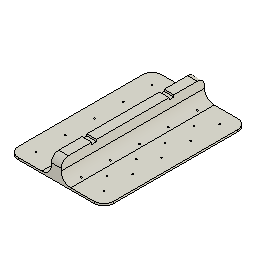
Tempeh-mould-10x15 (Autodesk Fusion 360 archive; units mm, degrees)
design "Tempeh-mould-lid-10x15"
Autodesk Fusion 360 part; units mm, degrees
sketch "sketch-footprint-box" plane through (0, 0, 0) normal (0, 0, 1) x (1, 0, 0)
  line L0 (-50, 75) -> (50, 75) construction
  line L1 (50, 75) -> (50, -75) construction
  line L2 (50, -75) -> (-50, -75) construction
  line L3 (-50, -75) -> (-50, 75) construction
  line L4 (-50, 75) -> (50, -75) construction
  line L5 (50, 75) -> (-50, -75) construction
  line L6 (49.25, 74.25) -> (-49.25, 74.25)
  line L7 (-49.25, 74.25) -> (-49.25, -74.25)
  line L8 (-49.25, -74.25) -> (49.25, -74.25)
  line L9 (49.25, -74.25) -> (49.25, 74.25)
  line L10 (49.25, 74.25) -> (-49.25, -74.25) construction
  line L11 (-49.25, 74.25) -> (49.25, -74.25) construction
  dimension "width" = 100
  dimension "length" = 150
  dimension "d104" = 0.75
  dimension "d105" = 0.75
  constraint horizontal L0
  constraint vertical L1
  constraint horizontal L2
  constraint vertical L3
  constraint midpoint L5 origin
  constraint horizontal L6
  constraint perpendicular L6 L7
  constraint parallel L6 L8
  constraint parallel L7 L9
  constraint coincident L10 origin
  constraint coincident L11 origin
  measures "width" distance of L0.start L0.end
  measures "length" distance of L0.start L2.end
  measures "d104" distance of L0 L6
  measures "d105" distance of L3 L7
extrude "Extrude1" add sketch "sketch-footprint-box" along normal blind 2
sketch "Sketch-lid" plane through (0, 0, 2) normal (0, 0, 1) x (-1, 0, 0)
  line L0 (5, -74.25) -> (-5, -74.25)
  line L1 (-5, -74.25) -> (-5, 74.25)
  line L2 (-5, 74.25) -> (5, 74.25)
  line L3 (5, 74.25) -> (5, -74.25)
  line L4 (5, -74.25) -> (-5, 74.25) construction
  line L5 (-5, -74.25) -> (5, 74.25) construction
  line L6 (-49.25, 74.25) -> (-49.25, -74.25)
  line L7 (-49.25, -74.25) -> (49.25, -74.25)
  line L8 (49.25, -74.25) -> (49.25, 74.25)
  line L9 (49.25, 74.25) -> (-49.25, 74.25)
  dimension "handle_width" = 10
  constraint horizontal L0
  constraint vertical L1
  constraint horizontal L2
  constraint vertical L3
  constraint midpoint L5 origin
  constraint coincident L1.end L9
  measures "handle_width" distance of L0.start L0.end
extrude "Extrude2" add sketch "Sketch-lid" along normal blind 20 contours L0 L1 L2 L3 L7 L9
extrude "Extrude8" add 1 faces at (16.4167, 24.75, 0) along direction (0, 0, -1) blind 0.0001
draft "Draft18" angle 0 neutral plane through (0, 0, 22) pull (0, 0, 1) 1 faces at (-5, -24.75, 8.6667)
draft "Draft19" angle 0 neutral plane through (0, 0, 22) pull (0, 0, 1) 1 faces at (5, 24.75, 8.6667)
draft "Draft20" angle 0 neutral plane through (0, 0, 22) pull (0, 0, 1) 1 faces at (-1.6667, -74.25, 8.6667)
draft "Draft21" angle 0 neutral plane through (0, 0, 22) pull (0, 0, 1) 1 faces at (1.6667, 74.25, 15.3333)
draft "Draft22" angle 0 neutral plane through (0, 0, 2) pull (0, 0, 1) 1 faces at (49.25, 24.75, 0.6666)
draft "Draft23" angle 0 neutral plane through (0, 0, 2) pull (0, 0, 1) 1 faces at (-49.25, 24.75, 1.3333)
fillet "Fillet5" radius 10 4 edges at (49.25, -74.25, 0.9999) (49.25, 74.25, 1) (-49.25, 74.25, 1) (-49.25, -74.25, 1)
fillet "Fillet6" radius 10 2 edges at (-5, 0, 2) (5, 0, 2)
fillet "Fillet7" radius 7.5 2 edges at (0, -74.25, 22) (0, 74.25, 22)
sketch "Sketch-notches-handle" plane through (0, 0, 22) normal (0, 0, 1) x (-1, 0, 0)
  line L0 (5, -66.75) -> (5, 66.75)
  line L1 (-5, 66.75) -> (-5, -66.75)
  line L2 (5, -42.5) -> (-5, -42.5)
  line L3 (-5, -42.5) -> (-5, -37.5)
  line L4 (-5, -37.5) -> (5, -37.5)
  line L5 (5, -37.5) -> (5, -42.5)
  line L6 (5, 37.5) -> (-5, 37.5)
  line L7 (-5, 37.5) -> (-5, 42.5)
  line L8 (-5, 42.5) -> (5, 42.5)
  line L9 (5, 42.5) -> (5, 37.5)
  line L10 (5, -37.5) -> (-5, 37.5) construction
  line L11 (-5, -37.5) -> (5, 37.5) construction
  line L12 (5, -37.5) -> (-5, -42.5) construction
  line L13 (5, -42.5) -> (-5, -37.5) construction
  line L14 (5, 42.5) -> (-5, 37.5) construction
  line L15 (-5, 42.5) -> (5, 37.5) construction
  circle A0 centre (0, -40) radius 0.75
  circle A1 centre (0, 40) radius 0.75
  line L16 (0, -37.5) -> (0, 0) construction
  line L17 (0, 0) -> (0, 37.5) construction
  line L18 (-5, -66.75) -> (5, -66.75)
  line L19 (5, 66.75) -> (-5, 66.75)
  dimension "handle_pocket" = 5
  dimension "d29" = 5
  dimension "hole_diameter" = 1.5
  dimension "d48" = 1.5
  dimension "d79" = 75
  constraint horizontal L2
  constraint vertical L3
  constraint horizontal L4
  constraint vertical L5
  constraint coincident L1 L3.end
  constraint coincident L0 L2.start
  constraint horizontal L6
  constraint vertical L7
  constraint horizontal L8
  constraint vertical L9
  constraint coincident L1 L7.end
  constraint coincident L0 L6.start
  constraint midpoint L10 L16.end
  constraint coincident L16.end L17.start
  constraint midpoint L13 A0.centre
  constraint midpoint L15 A1.centre
  constraint midpoint L4 L16.start
  constraint midpoint L6 L17.end
  measures "handle_pocket" distance of L2.start L4.end
  measures "d29" distance of L6.start L8.end
  measures "hole_diameter" diameter of A0
  measures "d48" diameter of A1
  measures "d79" distance of L3.end L6.end
extrude "Extrude3" cut sketch "Sketch-notches-handle" against normal blind 2 contours L0 L1 L2 L3 L4 L5 | L0 L1 L6 L7 L8 L9 | A0 | A1
sketch "Sketch-holes" plane through (0, 0, 2) normal (0, 0, 1) x (-1, 0, 0)
  line L0 (-50, -75) -> (50, -75) construction
  line L1 (50, -75) -> (50, 75) construction
  line L2 (50, 75) -> (-50, 75) construction
  line L3 (-50, 75) -> (-50, -75) construction
  line L4 (-50, -75) -> (50, 75) construction
  line L5 (50, -75) -> (-50, 75) construction
  line L6 (-35, -60) -> (35, -60) construction
  line L7 (35, -60) -> (35, 60) construction
  line L8 (35, 60) -> (-35, 60) construction
  line L9 (-35, 60) -> (-35, -60) construction
  circle A0 centre (35, -60) radius 0.75
  circle A1 centre (23.3333, -45) radius 0.75
  circle A2 centre (35, 30) radius 0.75
  line L10 (15, -74.25) -> (39.25, -74.25)
  line L11 (49.25, -64.25) -> (49.25, 64.25)
  line L12 (39.25, 74.25) -> (15, 74.25)
  line L13 (-49.25, 64.25) -> (-49.25, -64.25)
  line L14 (15, 74.25) -> (15, -74.25)
  line L15 (-15, -74.25) -> (-15, 74.25)
  line L16 (-15, 74.25) -> (-39.25, 74.25)
  line L17 (-39.25, -74.25) -> (-15, -74.25)
  circle A3 centre (-11.6667, -30) radius 0.75
  circle A4 centre (-11.6667, 30) radius 0.75
  circle A5 centre (35, -30) radius 0.75
  circle A6 centre (35, 0) radius 0.75
  circle A7 centre (23.3333, 15) radius 0.75
  circle A8 centre (-11.6667, -60) radius 0.75
  arc A9 (-39.25, 74.25) -> (-49.25, 64.25) centre (-39.25, 64.25) ccw
  arc A10 (-49.25, -64.25) -> (-39.25, -74.25) centre (-39.25, -64.25) ccw
  arc A11 (39.25, -74.25) -> (49.25, -64.25) centre (39.25, -64.25) ccw
  arc A12 (49.25, 64.25) -> (39.25, 74.25) centre (39.25, 64.25) ccw
  circle A13 centre (-35, -60) radius 0.75
  circle A14 centre (11.6667, -30) radius 0.75
  circle A15 centre (-35, -30) radius 0.75
  circle A16 centre (-23.3333, -15) radius 0.75
  circle A17 centre (11.6667, 0) radius 0.75
  circle A18 centre (-35, 0) radius 0.75
  circle A19 centre (-23.3333, 15) radius 0.75
  circle A20 centre (11.6667, 30) radius 0.75
  circle A21 centre (-35, 30) radius 0.75
  circle A22 centre (23.3333, 45) radius 0.75
  circle A23 centre (-23.3333, 45) radius 0.75
  circle A24 centre (35, 60) radius 0.75
  circle A25 centre (11.6667, 60) radius 0.75
  circle A26 centre (-11.6667, 60) radius 0.75
  circle A27 centre (-35, 60) radius 0.75
  circle A28 centre (11.6667, -60) radius 0.75
  circle A29 centre (23.3333, -15) radius 0.75
  circle A30 centre (-11.6667, 0) radius 0.75
  circle A31 centre (-23.3333, -45) radius 0.75
  dimension "d52" = 100
  dimension "d53" = 150
  dimension "hole_offset" = -15
  dimension "d55" = 1.5
  dimension "width_holes_surface" = -70
  dimension "length_holes_surface" = 120
  constraint horizontal L0
  constraint perpendicular L0 L1
  constraint parallel L0 L2
  constraint parallel L1 L3
  constraint coincident L4 origin
  constraint coincident L5 origin
  constraint coincident L6.end L7.start
  measures "d52" distance of L1.end L2.end
  measures "d53" distance of L0.end L1.end
  measures "d55" diameter of A0
extrude "Extrude7" cut sketch "Sketch-holes" along normal mid plane 30 contours A0 | A1 | A2 | A3 | A4 | A5 | A6 | A7 | A8 | A13 | A14 | A15 | A16 | A17 | A18 | A19 | A20 | A21 | A22 | A23 | A24 | A25 | A26 | A27 | A28 | A29 | A30 | A31
equation "thickness = 2 mm"
equation "handle_heigth = 20 mm"
equation "draft = 0 deg"
equation "corner_fillet = 10.00 mm"
equation "handle_end_fillet = 7.5 mm"
equation "handle_base_fillet = 10 mm"
equation "d29 = handle_pocket"
equation "handle_pocket_depth = -2.00 mm"
equation "mini_fillet = 1 mm"
equation "d48 = hole_diameter"
equation "hole_depth = -37.00 mm"
equation "d52 = width"
equation "d53 = length"
equation "d55 = hole_diameter"
equation "width_holes_number = 7" comment "width / 20 +2"
equation "length_holes_number = 9" comment "length / 20 + 2"
equation "width_holes_surface = -width - 2 * hole_offset"
equation "length_holes_surface = length + 2 * hole_offset"
equation "extra_bottom_thickness = 0.0001 mm"
equation "d79 = length / 2"
equation "width_offset = 0.75 mm"
equation "length_offset = 0.75 mm"
equation "d84 = draft"
equation "d86 = draft"
equation "d88 = draft"
equation "d90 = draft"
equation "d92 = draft"
equation "d94 = draft"
equation "d97 = corner_fillet"
equation "d99 = handle_base_fillet"
equation "d101 = handle_end_fillet"
equation "d104 = width_offset"
equation "d105 = length_offset"
named bodies: "lid"
